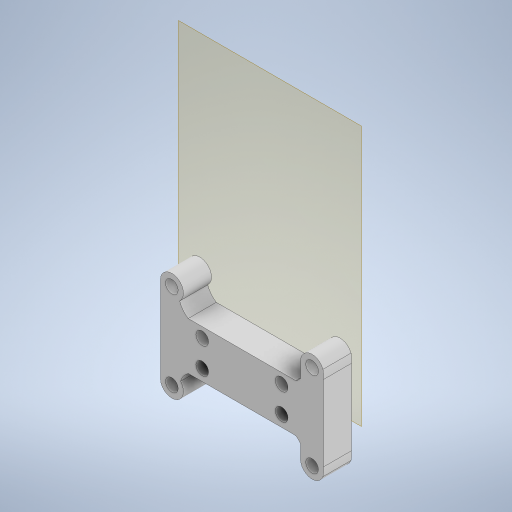
# Autodesk Inventor part: _arm_adt
Saved by Autodesk Inventor 2024.3 (Build 283343000, 343)
## iProperties
Created: 2024-09-06
Part Number: _arm_adt
Material: 일반
Document SubType Name: Modeling
Designer: gretc
Density: 1 g/cm^3
Appearance: 기본값
Author: gretc
Autodesk Inventor part; units mm, degrees
ref_plane "YZ Plane" through (0, 0, 0) normal (1, 0, 0) x (0, 1, 0)
ref_plane "XZ Plane" through (0, 0, 0) normal (0, 1, 0) x (-1, 0, 0)
ref_plane "XY Plane" through (0, 0, 0) normal (0, 0, 1) x (1, 0, 0)
ref_plane "작업 평면1" through (0, 0, 0) normal (0, 0, 1) x (1, 0, 0)
sketch "스케치1" plane through (0, 0, 0) normal (0, 0, 1) x (1, 0, 0)
  line L0 (12.7, -89.2) -> (9.2, -89.2) projected
  line L1 (12.7, -89.2) -> (17.8, -83.2) projected
  line L2 (17.8, -83.2) -> (17.8, -44.6) projected
  line L3 (17.8, -44.6) -> (12.7, -38.6) projected
  line L4 (12.7, -38.6) -> (-12.7, -38.6) projected
  line L5 (-12.7, -38.6) -> (-17.8, -44.6) projected
  line L6 (-17.8, -44.6) -> (-17.8, -83.2) projected
  line L7 (-17.8, -83.2) -> (-12.7, -89.2) projected
  line L8 (-9.2, -89.2) -> (-12.7, -89.2) projected
  arc A0 (-12.2, -86.2) -> (-9.2, -89.2) centre (-9.2, -86.2) ccw projected
  line L9 (-12.2, -47.2) -> (-12.2, -86.2) projected
  arc A1 (-9.2, -44.2) -> (-12.2, -47.2) centre (-9.2, -47.2) ccw projected
  line L10 (9.2, -44.2) -> (-9.2, -44.2) projected
  arc A2 (12.2, -47.2) -> (9.2, -44.2) centre (9.2, -47.2) ccw projected
  line L11 (12.2, -86.2) -> (12.2, -47.2) projected
  arc A3 (9.2, -89.2) -> (12.2, -86.2) centre (9.2, -86.2) ccw projected
  circle A4 centre (15, -81.7) radius 1.35 projected
  circle A5 centre (15, -64.7) radius 1.35 projected
  circle A6 centre (8.5, -41.4) radius 1.35 projected
  circle A7 centre (-15, -81.7) radius 1.35 projected
  circle A8 centre (-15, -64.7) radius 1.35 projected
  circle A9 centre (-8.5, -41.4) radius 1.35 projected
  circle A10 centre (15, -47.7) radius 1.35 projected
  circle A11 centre (-15, -47.7) radius 1.35 projected
  line L12 (-12.7, 12) -> (-9.2, 12) projected
  line L13 (-12.7, 12) -> (-17.8, 6) projected
  line L14 (-17.8, 6) -> (-17.8, -32.6) projected
  line L15 (-17.8, -32.6) -> (-12.7, -38.6) projected
  line L16 (-12.7, -38.6) -> (12.7, -38.6) projected
  line L17 (12.7, -38.6) -> (17.8, -32.6) projected
  line L18 (17.8, -32.6) -> (17.8, 6) projected
  line L19 (17.8, 6) -> (12.7, 12) projected
  line L20 (9.2, 12) -> (12.7, 12) projected
  arc A12 (12.2, 9) -> (9.2, 12) centre (9.2, 9) ccw projected
  line L21 (12.2, -30) -> (12.2, 9) projected
  arc A13 (9.2, -33) -> (12.2, -30) centre (9.2, -30) ccw projected
  line L22 (-9.2, -33) -> (9.2, -33) projected
  arc A14 (-12.2, -30) -> (-9.2, -33) centre (-9.2, -30) ccw projected
  line L23 (-12.2, 9) -> (-12.2, -30) projected
  arc A15 (-9.2, 12) -> (-12.2, 9) centre (-9.2, 9) ccw projected
  circle A16 centre (-15, 4.5) radius 1.35 projected
  circle A17 centre (-15, -12.5) radius 1.35 projected
  circle A18 centre (-8.5, -35.8) radius 1.35 projected
  circle A19 centre (15, 4.5) radius 1.35 projected
  circle A20 centre (15, -12.5) radius 1.35 projected
  circle A21 centre (8.5, -35.8) radius 1.35 projected
  circle A22 centre (-15, -29.5) radius 1.35 projected
  circle A23 centre (15, -29.5) radius 1.35 projected
  line L24 (-8.5, -43.8367) -> (-8.5, -33.6588)
  line L25 (-8.5, -33.6588) -> (8.5, -33.6588)
  line L26 (8.5, -33.6588) -> (8.5, -43.8367)
  line L27 (8.5, -43.8367) -> (-8.5, -43.8367)
  line L28 (-8.5, -43.8367) -> (-8.5, -33.6588)
  line L29 (-8.5, -33.6588) -> (-11.5, -33.6588)
  line L30 (-11.5, -33.6588) -> (-11.5, -43.8367)
  line L31 (-11.5, -43.8367) -> (-8.5, -43.8367)
  line L32 (8.5, -43.8367) -> (8.5, -33.6588)
  line L33 (8.5, -33.6588) -> (11.5, -33.6588)
  line L34 (11.5, -33.6588) -> (11.5, -43.8367)
  line L35 (11.5, -43.8367) -> (8.5, -43.8367)
  circle A24 centre (15, -47.7) radius 2.8
  circle A25 centre (15, -29.5) radius 2.8
  circle A26 centre (-15, -47.7) radius 2.8
  circle A27 centre (-15, -29.5) radius 2.8
  line L36 (17.8, -50.175) -> (13.5711, -50.175) projected
  line L37 (13.5711, -27.025) -> (17.8, -27.025) projected
  line L38 (-13.5711, -50.175) -> (-17.8, -50.175) projected
  line L39 (-17.8, -27.025) -> (-13.5711, -27.025) projected
  circle A28 centre (15, -47.7) radius 2.475
  circle A29 centre (15, -29.5) radius 2.475
  circle A30 centre (-15, -47.7) radius 2.475
  circle A31 centre (-15, -29.5) radius 2.475
  line L40 (15, -29.5) -> (11.5, -29.5)
  line L41 (12.525, -29.5) -> (12.525, -47.7)
  line L42 (12.525, -47.7) -> (12.525, -49.0093)
  line L43 (12.525, -29.5) -> (12.525, -28.1907)
  circle A32 centre (9.2, -47.2) radius 4.0745
  circle A33 centre (9.2, -30) radius 4.3217
  circle A34 centre (9.2, -47.2) radius 8.2366
  circle A35 centre (9.2, -30) radius 8.2366
  circle A36 centre (-9.2, -47.2) radius 8.2366
  circle A37 centre (-9.2, -30) radius 8.2439
  circle A38 centre (-9.2, -47.2) radius 4.0745
  circle A39 centre (-9.2, -30) radius 4.3217
  point P0 (0, 0)
  point P1 (-13.3169, -31.3146)
  point P2 (-17.3396, -28.6926)
  point P3 (-15.7015, -35.0688)
  point P4 (-15.25, -35.6)
  point P5 (-11.5, -37.9166)
  point P6 (-11.5, -39.2911)
  point P7 (-17.3258, -48.5464)
  point P8 (-13.1204, -46.0899)
  point P9 (12.525, -44.845)
  point P10 (17.3258, -48.5464)
  point P11 (12.525, -39.6644)
  point P12 (12.525, -37.5356)
  point P13 (17.3258, -28.6536)
  point P14 (12.525, -32.7607)
  dimension "d0" = 3
  dimension "d1" = 3
  constraints: 32 end point, 16 coincident, 9 centre point, 8 tangent, 6 parallel, 5 perpendicular, 4 point on line, 4 vertical, 2 horizontal, 2 point on circle, 21 other
  measures "d0" distance of L29.end L24.end
  measures "d1" distance of L25.end L33.end
extrude "돌출2" add sketch "스케치1" along normal blind 6 contours A34 A28 A32 A24 | A24 A32 L41 A34 | A34 L26 A6 A32 L27 | L27 A36 L24 L4 L26 A34 | A32 A28 L41 A24 | A24 L41 A32 | A28 A32 A34 | A32 L26 L27 | A28 A32 | L27 A38 L24 A9 A36 | A34 L34 A32 L26 A6 | L26 L4 L34 A34 | A34 L34 L4 L41 | L41 A32 L34 A34 | L26 A32 L35 | L27 L24 A38 | A36 L30 L4 L24 | L24 A9 A38 L30 A36 | L26 A35 L34 L4 | L4 L24 A37 L25 A35 L26 | L4 L34 A35 L41 | A35 L41 A33 A25 | L31 A38 L24 | L4 L30 A37 L24 | L30 A38 A26 A36 | A35 L25 A33 L26 A21 | L26 A21 A33 L34 A35 | A35 L34 A33 L41 | A25 A33 A29 A35 | A37 L30 A39 L24 A18 | L24 A18 A39 L25 A37 | L41 A25 A33 | A25 L41 A29 A33 | A38 A30 A36 A26 | A38 A30 | A30 A36 A38 | A37 L15 A27 A39 L30 | A33 L26 L33 | L25 L26 A33 | A33 A29 A35 | A29 L40 A33 | L29 L24 A39 | A39 L24 L25 | A29 A33 L40 | A27 A37 A31 A39 | A39 A31 | A31 A37 A39
sketch "스케치2" plane through (0, 0, 6) normal (0, 0, 1) x (1, 0, 0)
  line L0 (11.5, -33.6588) -> (-11.5, -33.6588) projected
  arc A0 (-13.3169, -31.3146) -> (-11.5, -33.6588) centre (-9.2, -30) ccw projected
  arc A1 (-13.3169, -31.3146) -> (-17.3396, -28.6926) centre (-15, -29.5) ccw projected
  arc A2 (-17.3396, -28.6926) -> (-15.7015, -35.0688) centre (-9.2, -30) ccw projected
  line L1 (-15.7015, -35.0688) -> (-15.25, -35.6) projected
  arc A3 (-15.25, -35.6) -> (-11.5, -37.9166) centre (-9.2, -30) ccw projected
  line L2 (-11.5, -37.9166) -> (-11.5, -39.2911) projected
  arc A4 (-11.5, -39.2911) -> (-17.3258, -48.5464) centre (-9.2, -47.2) ccw projected
  arc A5 (-17.3258, -48.5464) -> (-13.1204, -46.0899) centre (-15, -47.7) ccw projected
  arc A6 (-11.5, -43.8367) -> (-13.1204, -46.0899) centre (-9.2, -47.2) ccw projected
  line L3 (-11.5, -43.8367) -> (11.5, -43.8367) projected
  arc A7 (12.525, -44.845) -> (11.5, -43.8367) centre (9.2, -47.2) ccw projected
  line L4 (12.525, -44.845) -> (12.525, -47.7) projected
  arc A8 (12.525, -47.7) -> (17.3258, -48.5464) centre (15, -47.7) ccw projected
  arc A9 (17.3258, -48.5464) -> (12.525, -39.6644) centre (9.2, -47.2) ccw projected
  line L5 (12.525, -39.6644) -> (12.525, -37.5356) projected
  arc A10 (12.525, -37.5356) -> (17.3258, -28.6536) centre (9.2, -30) ccw projected
  arc A11 (17.3258, -28.6536) -> (12.525, -29.5) centre (15, -29.5) ccw projected
  line L6 (12.525, -29.5) -> (12.525, -32.7607) projected
  arc A12 (11.5, -33.6588) -> (12.525, -32.7607) centre (9.2, -30) ccw projected
  circle A13 centre (15, -47.7) radius 1.35 projected
  circle A14 centre (8.5, -35.8) radius 1.35 projected
  circle A15 centre (15, -29.5) radius 1.35 projected
  circle A16 centre (8.5, -41.4) radius 1.35 projected
  circle A17 centre (-8.5, -41.4) radius 1.35 projected
  circle A18 centre (-15, -47.7) radius 1.35 projected
  circle A19 centre (-15, -29.5) radius 1.35 projected
  circle A20 centre (-8.5, -35.8) radius 1.35 projected
  line L7 (-17.4288, -29.5) -> (17.4214, -29.5)
  line L8 (-15, -47.7) -> (17.4214, -47.7)
  line L9 (-15, -47.7) -> (-18, -47.7)
  line L10 (-15, -47.7) -> (-12, -47.7) construction
  line L11 (17.4214, -29.5) -> (17.4214, -47.7)
  line L12 (17.4214, -47.7) -> (-17.4288, -47.7)
  line L13 (-17.4288, -47.7) -> (-17.4288, -29.5)
  line L14 (-17.4288, -29.5) -> (17.4214, -29.5)
  point P0 (0, 0)
  point P1 (17.4214, -46.7)
  point P2 (17.4214, -30.5)
  point P3 (-17.4288, -30.5)
  point P4 (-17.4288, -46.8415)
  dimension "d6" = 3
  dimension "d7" = 180
  constraints: 16 end point, 3 horizontal, 3 point on circle, 2 collinear, 2 parallel, 1 perpendicular, 1 vertical
  measures "d6" distance of L8.start L9.end
  measures "d7" angle of L9 L10
extrude "돌출3" add sketch "스케치2" against normal blind 6 contours L11 A9 L5 A10 | A2 L1 A3 L2 A4 L13
